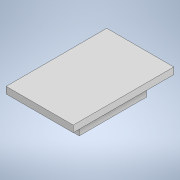
# Autodesk Inventor part: Part1
Saved by Autodesk Inventor 2022 (Build 260153000, 153)
## iProperties
Created: 2022-04-20
Part Number: Part1
Material: Generic
Document SubType Name: Modeling
Designer: Fred
Density: 1 g/cm^3
Appearance: Default
Author: Fred
Autodesk Inventor part; units mm, degrees
ref_plane "YZ Plane" through (0, 0, 0) normal (1, 0, 0) x (0, 1, 0)
ref_plane "XZ Plane" through (0, 0, 0) normal (0, 1, 0) x (-1, 0, 0)
ref_plane "XY Plane" through (0, 0, 0) normal (0, 0, 1) x (1, 0, 0)
sketch "Sketch1" plane through (0, 0, 0) normal (0, 1, 0) x (-1, 0, 0)
  line L0 (0, 0) -> (14, 0)
  line L1 (14, 0) -> (14, -8.4)
  line L2 (14, -8.4) -> (0, -8.4)
  line L3 (0, -8.4) -> (0, 0)
  dimension "d0" = 8.4
  dimension "d1" = 14
  constraints: 8 end point, 2 parallel, 1 coincident, 1 horizontal, 1 perpendicular
  measures "d0" distance of L0.end L1.end
  measures "d1" distance of L1.end L2.end
extrude "Extrusion1" add sketch "Sketch1" along normal blind 2.5
sketch "Sketch2" plane through (0, 2.5, 0) normal (0, 1, 0) x (1, 0, 0)
  line L0 (-14, 2.85) -> (-5, 2.85)
  line L1 (-5, 5.55) -> (-14, 5.55)
  line L2 (-14, 5.55) -> (-14, 2.85)
  line L3 (-14, 8.4) -> (-14, 0) projected
  line L4 (-5, 2.85) -> (-5, 0)
  line L5 (-14, 0) -> (0, 0) projected
  line L6 (-5, 0) -> (0, 0)
  line L7 (0, 0) -> (0, 8.4) projected
  line L8 (0, 0) -> (0, 8.4)
  line L9 (-5, 5.55) -> (-5, 8.4)
  line L10 (0, 8.4) -> (-14, 8.4) projected
  point P0 (-14, 4.2)
  point P1 (-14, 4.2)
  point P2 (-5, 1.425)
  point P3 (-5, 6.975)
  dimension "d4" = 9
  constraints: 14 end point, 5 midpoint, 3 vertical, 2 point on line, 1 coincident, 1 collinear, 1 horizontal, 1 parallel, 1 vertical alignment
  measures "d4" distance of L1.start L1.end
extrude "Extrusion2" add sketch "Sketch2" along normal blind 10 contours L2 L1 L9 L10 L7 L5 L4 L0
sketch "Sketch3" plane through (0, 0, 0) normal (0, -1, 0) x (1, 0, 0)
  line L0 (0, -29.6) -> (8, -29.6)
  line L1 (8, -29.6) -> (8, 21.2)
  line L2 (8, 21.2) -> (0, 21.2)
  line L3 (0, 21.2) -> (0, -29.6)
  line L4 (0, 0) -> (0, -8.4) projected
  point P0 (8, -4.2)
  point P1 (0, -4.2)
  point P2 (0, -4.2)
  dimension "d8" = 50.8
  dimension "d9" = 8
  constraints: 8 end point, 4 midpoint, 2 parallel, 1 horizontal, 1 horizontal alignment, 1 perpendicular
  measures "d8" distance of L0.end L1.end
  measures "d9" distance of L0.start L0.end
extrude "Extrusion3" add sketch "Sketch3" against normal up to surface (12.5 mm away)
sketch "Sketch4" plane through (0, 12.5, 0) normal (0, 1, 0) x (1, 0, 0)
  line L0 (16.1115, -33.9) -> (-34.6885, -33.9)
  line L1 (-34.6885, -33.9) -> (-34.6885, 42.3)
  line L2 (-34.6885, 42.3) -> (16.1115, 42.3)
  line L3 (16.1115, 42.3) -> (16.1115, -33.9)
  line L4 (8, 29.6) -> (8, -21.2) projected
  point P0 (0, 0)
  point P1 (16.1115, 4.2)
  point P2 (8, 4.2)
  dimension "d12" = 50.8
  dimension "d13" = 76.2
  constraints: 8 end point, 2 midpoint, 2 parallel, 1 horizontal, 1 horizontal alignment, 1 perpendicular
  measures "d12" distance of L0.start L0.end
  measures "d13" distance of L0.end L1.end
extrude "Extrusion4" add sketch "Sketch4" along normal blind 5
body "Solid1"
